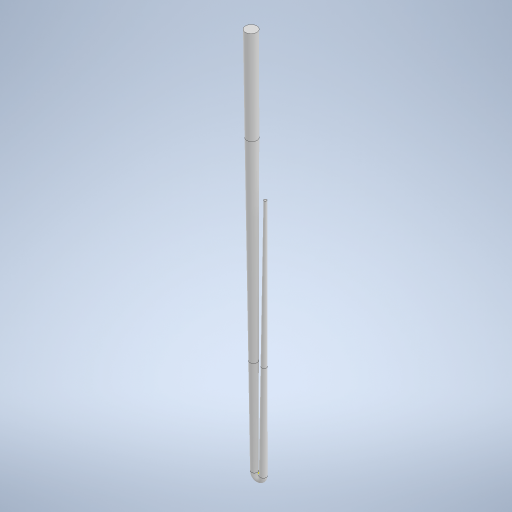
# Autodesk Inventor part: bore
Saved by Autodesk Inventor 2023 (Build 270158000, 158)
## iProperties
Created: 2023-02-09
Part Number: bore
Material: Generic
Document SubType Name: Modeling
Designer: dncob
Density: 1 g/cm^3
Appearance: Default
Author: dncob
Autodesk Inventor part; units mm, degrees
ref_plane "YZ Plane" through (0, 0, 0) normal (1, 0, 0) x (0, 1, 0)
ref_plane "XZ Plane" through (0, 0, 0) normal (0, 1, 0) x (-1, 0, 0)
ref_plane "XY Plane" through (0, 0, 0) normal (0, 0, 1) x (1, 0, 0)
sketch "bore path" plane through (0, 0, 0) normal (0, 0, 1) x (1, 0, 0)
  line L0 (22.045, 812.9386) -> (17.7602, 321.9573)
  line L1 (-26.2163, 1290.9204) -> (-23.45, 973.9344)
  arc A0 (-14.9494, -0.1305) -> (14.9494, -0.1305) centre (0, 0) ccw
  line L2 (0, 0) -> (0, 156.1202) construction
  line L3 (22.045, 812.9386) -> (26.495, 812.8997)
  line L4 (26.495, 812.8997) -> (26.0102, 321.8853)
  line L5 (17.7602, 321.9573) -> (26.0102, 321.8853) construction
  line L6 (17.7602, 321.9573) -> (14.9494, -0.1305)
  line L7 (26.0102, 321.8853) -> (25.399, -0.2217)
  line L8 (-30.4098, 321.8489) -> (-25.399, -0.2217)
  line L9 (-30.4098, 321.8489) -> (-17.7603, 321.9593) construction
  line L10 (-24.085, 321.9041) -> (-24.0265, 315.1961) construction
  line L11 (14.9494, -0.1305) -> (25.399, -0.2217) construction
  line L12 (-14.9494, -0.1305) -> (-25.399, -0.2217) construction
  line L13 (20.1742, -0.1761) -> (20.1742, 3.9012) construction
  line L14 (-17.7603, 321.9593) -> (-14.9494, -0.1305)
  line L15 (-20.1742, -0.1761) -> (-19.9393, -27.0948) construction
  arc A1 (-25.399, -0.2217) -> (25.399, -0.2217) centre (0, 0) ccw
  line L16 (21.8852, 321.9213) -> (21.7783, 309.6646) construction
  line L17 (-45.6155, 1290.7511) -> (-26.2163, 1290.9204)
  line L18 (-30.4098, 321.8489) -> (-40.95, 973.7817)
  line L19 (-40.95, 973.7817) -> (-45.6155, 1290.7511)
  line L20 (-40.95, 973.7817) -> (-23.45, 973.9344) construction
  line L21 (-23.45, 973.9344) -> (-17.7603, 321.9593)
  dimension "d3" = 813.1
  dimension "d5" = 179
  dimension "d7" = 1291.1
  dimension "d8" = 491
  dimension "d9" = 4.45
  dimension "d10" = 8.25
  dimension "d13" = 12.65
  dimension "d14" = 322.102
  dimension "d18" = 25.4
  dimension "d20" = 10.45
  dimension "d22" = 652
  dimension "d23" = 17.5
  dimension "d25" = 19.4
  constraints: 44 end point, 12 perpendicular, 5 tangent, 4 midpoint, 4 point on circle, 2 centre point, 2 coincident, 1 vertical, 1 other
  measures "d3" distance of L0.start L6.end
  measures "d7" distance of L1.start L12.start
  measures "d8" distance of L0.start L0.end
  measures "d9" horizontal distance of L0.start L3.end
  measures "d10" horizontal distance of L0.end L4.end
  measures "d13" distance of L8.start L9.end
  measures "d14" distance of L9.end L12.start
  measures "d18" radius of A1
  measures "d20" distance of L6.end L7.end
  measures "d22" distance of L1.end L9.end
  measures "d23" horizontal distance of L18.end L1.end
  measures "d25" distance of L17.start L1.start
ref_plane "Work Plane2" through (22.045, 812.9386, 0) normal (-0.0087265, -0.9999619, 0) x (0.9999619, -0.0087265, 0)
sketch "tenor" plane through (22.045, 812.9386, 0) normal (-0.0087265, -0.9999619, 0) x (0.9999619, -0.0087265, 0)
  circle A0 centre (0, 0) radius 4.4502
  line L0 (0, 0) -> (4.4502, 0) projected
  constraints: 1 coincident, 1 horizontal alignment, 2 other
ref_plane "Work Plane3" through (21.8852, 321.9213, 0) normal (-0.0087265, -0.9999619, 0) x (0.9999619, -0.0087265, 0)
sketch "boot" plane through (21.8852, 321.9213, 0) normal (-0.0087265, -0.9999619, 0) x (0.9999619, -0.0087265, 0)
  circle A0 centre (-4.1252, 0) radius 8.2503
  line L0 (-4.1252, 0) -> (4.1252, 0) construction
  point P0 (-19.0752, 0)
  constraints: 1 coincident, 1 horizontal alignment, 2 other
ref_plane "Work Plane4" through (14.9494, -0.1305, 0) normal (-0.0087265, -0.9999619, 0) x (0.9999619, -0.0087265, 0)
sketch "turn entrance" plane through (14.9494, -0.1305, 0) normal (-0.0087265, -0.9999619, 0) x (0.9999619, -0.0087265, 0)
  circle A0 centre (0, 0) radius 10.45
  line L0 (0, 0) -> (10.45, 0) construction
  point P0 (-14.95, 0)
  constraints: 1 coincident, 1 horizontal alignment, 2 other
ref_plane "Work Plane5" through (-14.9494, -0.1305, 0) normal (0.0087265, -0.9999619, 0) x (0.9999619, 0.0087265, 0)
sketch "turn exit" plane through (-14.9494, -0.1305, 0) normal (0.0087265, -0.9999619, 0) x (0.9999619, 0.0087265, 0)
  circle A0 centre (0, 0) radius 10.45
  line L0 (0, 0) -> (-10.45, 0) construction
  point P0 (14.95, 0)
  constraints: 1 coincident, 1 horizontal alignment, 2 other
ref_plane "Work Plane6" through (-17.7603, 321.9593, 0) normal (0.0087265, -0.9999619, 0) x (0.9999619, 0.0087265, 0)
sketch "bass" plane through (-17.7603, 321.9593, 0) normal (0.0087265, -0.9999619, 0) x (0.9999619, 0.0087265, 0)
  circle A0 centre (0, 0) radius 12.65
  line L0 (-12.65, 0) -> (0, 0) construction
  point P0 (14.95, 0)
  constraints: 1 coincident, 1 horizontal alignment, 2 other
ref_plane "Work Plane7" through (-23.45, 973.9344, 0) normal (0.0087265, -0.9999619, 0) x (0.9999619, 0.0087265, 0)
sketch "bell" plane through (-23.45, 973.9344, 0) normal (0.0087265, -0.9999619, 0) x (0.9999619, 0.0087265, 0)
  circle A0 centre (0, 0) radius 17.5007
  line L0 (-17.5007, 0) -> (0, 0) construction
  point P0 (14.95, 0)
  constraints: 1 coincident, 1 horizontal alignment, 2 other
ref_plane "Work Plane8" through (-26.2163, 1290.9204, 0) normal (0.0087265, -0.9999619, 0) x (0.9999619, 0.0087265, 0)
sketch "bell exit" plane through (-26.2163, 1290.9204, 0) normal (0.0087265, -0.9999619, 0) x (0.9999619, 0.0087265, 0)
  circle A0 centre (0, 0) radius 19.4
  line L0 (-19.4, 0) -> (0, 0) projected
  point P0 (14.95, 0)
  constraints: 1 coincident, 1 horizontal alignment, 2 other
sketch "Sketch12" plane through (0, 0, 0) normal (0, 0, 1) x (1, 0, 0)
  point P0 (0, 0)
loft "tenor loft" add profiles "tenor", "boot"
loft "boot loft 1" add profiles "boot", "turn entrance"
loft "boot loft 3" add profiles "turn exit", "bass"
loft "bass loft" add profiles "bass", "bell"
loft "bell loft" add profiles "bell", "bell exit"
sketch "turn path" plane through (0, 0, 0) normal (0, 0, 1) x (1, 0, 0)
  arc A0 (-14.9494, -0.1305) -> (14.9494, -0.1305) centre (0, 0) ccw projected
  arc A1 (-14.95, 0) -> (14.95, 0) centre (0, 0) ccw
  line L0 (25.399, -0.2217) -> (4.4998, -0.0393) projected
  line L1 (0, 0) -> (14.95, 0)
  constraints: 2 end point, 2 point on circle, 1 centre point, 1 coincident, 1 concentric, 1 horizontal
sweep "turn" add profiles "turn entrance" path "turn path" path curves A0
body "Solid1"
